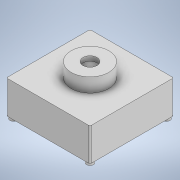
# Autodesk Inventor part: AERO - Base
Saved by Autodesk Inventor 2021 (Build 250183000, 183)
## iProperties
Created: 2021-01-21
Part Number: AERO - Base
Material: Generic
Document SubType Name: Modeling
Designer: garciar1
Density: 1 g/cm^3
Appearance: Default
Author: garciar1
Autodesk Inventor part; units mm, degrees
ref_plane "YZ Plane" through (0, 0, 0) normal (1, 0, 0) x (0, 1, 0)
ref_plane "XZ Plane" through (0, 0, 0) normal (0, 1, 0) x (-1, 0, 0)
ref_plane "XY Plane" through (0, 0, 0) normal (0, 0, 1) x (1, 0, 0)
sketch "Sketch1" plane through (0, 0, 0) normal (0, 1, 0) x (-1, 0, 0)
  line L0 (89, -89) -> (-89, -89)
  line L1 (-89, -89) -> (-89, 89)
  line L2 (-89, 89) -> (89, 89)
  line L3 (89, 89) -> (89, -89)
  point P0 (0, 0)
  dimension "d0" = 89
  dimension "d1" = 178
  dimension "d2" = 178
  dimension "d3" = 89
  constraints: 8 end point, 2 parallel, 1 horizontal, 1 perpendicular
  measures "d0" distance from line of L1 point (0, 0)
  measures "d1" distance of L0.start L0.end
  measures "d2" distance of L0.end L1.end
  measures "d3" distance from line of L0 point (0, 0)
extrude "Extrusion1" add sketch "Sketch1" along normal blind 70
sketch "Sketch2" plane through (0, 70, 0) normal (0, 1, 0) x (1, 0, 0)
  circle A0 centre (0, 0) radius 40
  dimension "d6" = 80
  constraints: 1 centre point, 1 coincident
  measures "d6" diameter of A0
extrude "Extrusion2" add sketch "Sketch2" along normal blind 30
sketch "Sketch3" plane through (0, 100, 0) normal (0, 1, 0) x (1, 0, 0)
  circle A0 centre (0, 0) radius 15
  dimension "d9" = 30
  constraints: 1 centre point, 1 coincident
  measures "d9" diameter of A0
extrude "Extrusion3" cut sketch "Sketch3" against normal blind 10
sketch "Sketch4" plane through (0, 0, 0) normal (0, -1, 0) x (1, 0, 0)
  circle A0 centre (-81.5, 81.5) radius 7.5
  line L0 (-89, 89) -> (89, 89) projected
  line L1 (-89, -89) -> (-89, 89) projected
  circle A1 centre (-81.5, -81.5) radius 7.5
  circle A2 centre (81.5, -81.5) radius 7.5
  circle A3 centre (81.5, 81.5) radius 7.5
  point P0 (0, 0)
  dimension "d12" = 15
  dimension "d13" = 7.5
  dimension "d14" = 7.5
  dimension "d17" = 360
  constraints: 4 centre point, 1 tangent, 9 other
  measures "d12" diameter of A0
  measures "d13" distance from line of L1 A0.centre
  measures "d14" distance from line of L0 A0.centre
extrude "Extrusion4" add sketch "Sketch4" along normal blind 5 contours A0 | A1 | A2 | A3
fillet "Fillet1" radius 3 4 edges at (-89, 35, 89) (89, 35, 89) (-89, 35, -89) (89, 35, -89)
body "Solid1"
